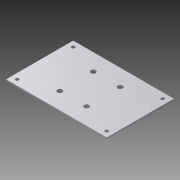
# Autodesk Inventor part: キャスター調節板
Saved by Autodesk Inventor 2015 (Build 190159000, 159)
## iProperties
Created: 2015-05-17
Part Number: キャスター調節板
Material: アルミニウム 6061
Document SubType Name: Modeling
Designer: kenta
Density: 2.7 g/cm^3
Appearance: アルミニウム - フラット - Version 1.1
Mass: 21.4901 g
Surface Area: 112.056 cm^2
Volume: 7.95929 cm^3
Author: kenta
Autodesk Inventor part; units mm, degrees
ref_plane "YZ Plane" through (0, 0, 0) normal (1, 0, 0) x (0, 1, 0)
ref_plane "XZ Plane" through (0, 0, 0) normal (0, 1, 0) x (-1, 0, 0)
ref_plane "XY Plane" through (0, 0, 0) normal (0, 0, 1) x (1, 0, 0)
sketch "スケッチ12" plane through (0, 0, 0) normal (0, 0, 1) x (1, 0, 0)
  line L0 (-45, 30) -> (45, 30)
  line L1 (45, 30) -> (45, -30)
  line L2 (45, -30) -> (-45, -30)
  line L3 (-45, -30) -> (-45, 30)
  line L4 (-45, 30) -> (45, -30) construction
  line L5 (45, 30) -> (-45, -30) construction
  point P0 (0, 0)
  dimension "d38" = 90
  dimension "d39" = 60
  constraints: 12 end point, 2 midpoint, 2 parallel, 1 horizontal, 1 perpendicular
  measures "d38" distance of L1.end L2.end
  measures "d39" distance of L0.end L1.end
extrude "押し出し5" add sketch "スケッチ12" along normal blind 1.5
sketch "スケッチ13" plane through (0, 0, 1.5) normal (0, 0, 1) x (1, 0, 0)
  line L0 (-45, 30) -> (-45, -30) projected
  line L1 (45, -30) -> (45, 30) projected
  line L2 (45, 30) -> (-45, 30) projected
  line L3 (-45, -30) -> (45, -30) projected
  point P0 (0, 0)
  point P1 (-40, 25)
  point P2 (-40, -25)
  point P3 (40, -25)
  point P4 (40, 25)
  dimension "d60" = 5
  dimension "d61" = 5
  dimension "d62" = 5
  dimension "d63" = 5
  constraints: 2 vertical alignment, 1 horizontal alignment
  measures "d60" distance from line of point (-40, 25) L0
  measures "d61" distance from line of point (40, 25) L1
  measures "d62" distance from line of point (40, 25) L2
  measures "d63" distance from line of point (40, -25) L3
hole "穴5" at (-40, 25, 1.5) at (-40, -25, 1.5) at (40, -25, 1.5) at (40, 25, 1.5) direction (0, 0, -1) diameter 3.1 end through all
sketch "スケッチ14" plane through (0, 0, 1.5) normal (0, 0, 1) x (1, 0, 0)
  point P0 (0, 0)
  point P1 (-12, 15)
  point P2 (12, 15)
  point P3 (-12, -15)
  point P4 (12, -15)
  dimension "d56" = 15
  dimension "d57" = 15
  dimension "d58" = 15
  dimension "d59" = 15
  dimension "d64" = 12
  dimension "d65" = 12
  dimension "d66" = 12
  dimension "d67" = 12
  measures "d56" vertical distance of point (-12, 15) point (0, 0)
  measures "d57" vertical distance of point (0, 0) point (12, 15)
  measures "d58" vertical distance of point (-12, -15) point (0, 0)
  measures "d59" vertical distance of point (12, -15) point (0, 0)
  measures "d64" horizontal distance of point (0, 0) point (12, 15)
  measures "d65" horizontal distance of point (0, 0) point (-12, 15)
  measures "d66" horizontal distance of point (0, 0) point (-12, -15)
  measures "d67" horizontal distance of point (0, 0) point (12, -15)
hole "穴6" at (-12, 15, 1.5) at (12, 15, 1.5) at (-12, -15, 1.5) at (12, -15, 1.5) direction (0, 0, -1) diameter 4.5 end through all
